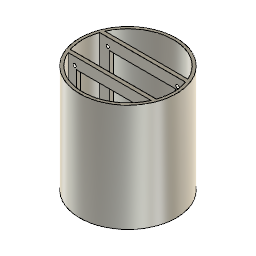
GeneralAvionicsMount (Autodesk Fusion 360 design; units mm, degrees)
Autodesk Fusion 360 part; units mm, degrees
sketch "Sketch1" plane through (0, 0, 0) normal (0, 0, 1) x (1, 0, 0)
  circle A0 centre (0, 0) radius 38.1
  circle A1 centre (0, 0) radius 35.814
  line L0 (0, 0) -> (0, -19.5613) construction
  line L1 (-30, -19.5613) -> (30, -19.5613)
  line L2 (30, -19.5613) -> (30, -14.5613) construction
  line L3 (30, -14.5613) -> (-30, -14.5613)
  line L4 (-30, -14.5613) -> (-30, -19.5613) construction
  line L5 (-30, -14.5613) -> (-32.7202, -14.5613)
  line L6 (30, -14.5613) -> (32.7202, -14.5613)
  line L7 (-33.8966, -11.5613) -> (33.8966, -11.5613)
  line L8 (-30, -19.5613) -> (-32.6951, -19.5613)
  line L9 (30, -19.5613) -> (32.6951, -19.5613)
  line L10 (-30.7018, -22.5613) -> (30.7018, -22.5613)
  line L11 (-30, 14.5613) -> (30, 14.5613)
  line L12 (30, 14.5613) -> (32.7202, 14.5613)
  line L13 (33.8966, 11.5613) -> (-33.8966, 11.5613)
  line L14 (30, 14.5613) -> (30, 19.5613) construction
  line L15 (-30, 19.5613) -> (-32.6951, 19.5613)
  line L16 (30, 19.5613) -> (32.6951, 19.5613)
  line L17 (-30, 19.5613) -> (-30, 14.5613) construction
  line L18 (30, 19.5613) -> (-30, 19.5613)
  line L19 (30.7018, 22.5613) -> (-30.7018, 22.5613)
  line L20 (-30, 14.5613) -> (-32.7202, 14.5613)
  point P0 (0, 19.5613)
  dimension "d1" = 76.2
  dimension "d2" = 71.628
  dimension "d10" = 5
  dimension "d11" = 60
  dimension "d12" = 3
  dimension "d13" = 3
  dimension "d15" = 360
  constraint coincident A0.centre A1.centre
  constraint concentric A0 A1
  constraint horizontal L1
  constraint vertical L2
  constraint horizontal L3
  constraint vertical L4
  constraint coincident A1 L1.start
  constraint coincident A1 L1.end
  constraint coincident A1 L5.end
  constraint perpendicular L4 L5
  constraint coincident A1 L6.end
  constraint perpendicular L2 L6
  constraint coincident A1 L7.start
  constraint coincident A1 L7.end
  constraint horizontal L7
  constraint coincident A0 L8.end
  constraint perpendicular L4 L8
  constraint coincident A0 L9.end
  constraint perpendicular L2 L9
  constraint coincident A0 L10.start
  constraint coincident A0 L10.end
  constraint horizontal L10
  measures "d1" diameter of A0
  measures "d2" diameter of A1
  measures "d10" distance of L1.start L3.end
  measures "d11" distance of L1.start L1.end
  measures "d12" distance of L3 L7
  measures "d13" distance of L1 L10
extrude "Extrude2" add sketch "Sketch1" along normal blind 85 contours A0 A1 L9 L16 | A0 A1 L16 L19 | A0 A1 L9 L10 | A0 A1 L19 | A0 A1 L10 | A0 A1 L15 L19 | A1 L11 L12 L13 L20 | A0 A1 L8 L15 | A0 A1 L8 L10 | A1 L3 L5 L6 L7
sketch "Sketch3" plane through (0, 14.5613, 0) normal (0, 1, 0) x (-1, 0, 0)
  line L0 (-32.7202, 0) -> (32.7202, 0)
  line L1 (32.7202, 0) -> (32.7202, 85)
  line L2 (32.7202, 85) -> (-32.7202, 85)
  line L3 (-32.7202, 85) -> (-32.7202, 0)
  line L4 (27.5, 6.25) -> (-27.5, 6.25) construction
  line L5 (-27.5, 6.25) -> (-27.5, 78.75) construction
  line L6 (-27.5, 78.75) -> (27.5, 78.75) construction
  line L7 (27.5, 78.75) -> (27.5, 6.25) construction
  line L8 (5.5903, 6.25) -> (5.5903, 0) construction
  line L9 (8.4326, 78.75) -> (8.4326, 85) construction
  line L10 (-32.7202, 48.7618) -> (-27.5, 48.7618) construction
  line L11 (32.7202, 50.3453) -> (27.5, 50.3453) construction
  circle A0 centre (27.5, 78.75) radius 1.625
  circle A1 centre (-27.5, 78.75) radius 1.625
  circle A2 centre (-27.5, 6.25) radius 1.625
  circle A3 centre (27.5, 6.25) radius 1.625
  line L12 (26, 8.5) -> (-26, 8.5)
  line L13 (-26, 8.5) -> (-26, 76.5)
  line L14 (-26, 76.5) -> (26, 76.5)
  line L15 (26, 76.5) -> (26, 8.5)
  line L16 (14.1085, 76.5) -> (14.1085, 78.75)
  line L17 (12.9666, 8.5) -> (12.9666, 6.25)
  line L18 (26, 26.5961) -> (27.5, 26.5961) construction
  line L19 (-26, 37.0362) -> (-27.5, 37.0362)
  line L20 (-26, 35.2418) -> (-27.5, 35.2418) construction
  dimension "d18" = 72.5
  dimension "d19" = 55
  dimension "d21" = 3.25
  dimension "d24" = 52
  dimension "d25" = 68
  constraint horizontal L4
  constraint vertical L5
  constraint horizontal L6
  constraint vertical L7
  constraint coincident L4 L8.start
  constraint coincident L0 L8.end
  constraint perpendicular L0 L8
  constraint coincident L6 L9.start
  constraint coincident L2 L9.end
  constraint perpendicular L2 L9
  constraint equal L8 L9
  constraint coincident L3 L10.start
  constraint coincident L5 L10.end
  constraint perpendicular L5 L10
  constraint coincident L1 L11.start
  constraint coincident L7 L11.end
  constraint perpendicular L7 L11
  constraint equal L10 L11
  constraint coincident L6.end L7.start
  constraint coincident L5.end L6.start
  constraint coincident L4.end L5.start
  constraint coincident L4.start L7.end
  constraint equal A2 A3
  constraint equal A1 A2
  constraint equal A0 A1
  constraint horizontal L12
  constraint vertical L13
  constraint horizontal L14
  constraint vertical L15
  constraint coincident L14 L16.start
  constraint coincident L6 L16.end
  constraint perpendicular L6 L16
  constraint coincident L12 L17.start
  constraint coincident L4 L17.end
  constraint perpendicular L4 L17
  constraint coincident L15 L18.start
  constraint coincident L7 L18.end
  constraint perpendicular L7 L18
  constraint coincident L13 L19.start
  constraint coincident L5 L19.end
  constraint perpendicular L5 L19
  constraint coincident L13 L20.start
  constraint coincident L5 L20.end
  constraint perpendicular L5 L20
  constraint equal L16 L17
  constraint equal L18 L20
  measures "d18" distance of L4.start L6.end
  measures "d19" distance of L4.start L4.end
  measures "d21" diameter of A0
  measures "d24" distance of L13.end L14.end
  measures "d25" distance of L12.end L13.end
extrude "Extrude3" cut sketch "Sketch3" against normal up to surface (29.1225 mm away) contours A0 | A1 | A2 | A3 | L12 L13 L14 L15
thread "Thread1" "ISO Metric profile 3.0 M3x0.5 M3x0.5 6H" major diameter 3.086 minor diameter 2.529 pitch 0.5 angle 60 resizes the face on face at (-26.8317, -12.5613, 80.2312) on face at (-26.8317, 12.5613, 80.2312) on face at (28.1683, -12.5613, 80.2312) on face at (28.1683, 12.5613, 80.2312)
thread "Thread2" "ISO Metric profile 3.0 M3x0.5 M3x0.5 6H" major diameter 3.086 minor diameter 2.529 pitch 0.5 angle 60 resizes the face on face at (25.8831, -12.5613, 6.0882) on face at (-29.1169, -12.5613, 6.0882) on face at (25.8831, 13.5613, 6.0882) on face at (-29.1169, 13.5613, 6.0882)
